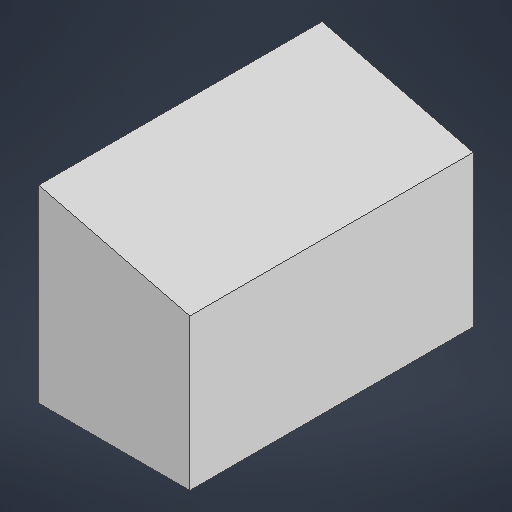
# Autodesk Inventor part: Housing og Buttons & LCD
Saved by Autodesk Inventor 2026.2 (Build 302298010, 298A)
## iProperties
Created: 2026-05-24
Part Number: Housing og Buttons & LCD
Material: Generic
Document SubType Name: Modeling
Designer: lenovo
Density: 1 g/cm^3
Appearance: Default
Author: lenovo
Autodesk Inventor part; units mm, degrees
ref_plane "YZ Plane" through (0, 0, 0) normal (1, 0, 0) x (0, 1, 0)
ref_plane "XZ Plane" through (0, 0, 0) normal (0, 1, 0) x (-1, 0, 0)
ref_plane "XY Plane" through (0, 0, 0) normal (0, 0, 1) x (1, 0, 0)
sketch "Sketch1" plane through (0, 0, 0) normal (0, 0, 1) x (1, 0, 0)
  line L0 (0, 0) -> (80, 0)
  line L1 (0, 0) -> (0, 100)
  line L2 (80, 0) -> (80, 80)
  line L3 (80, 80) -> (0, 100)
  dimension "d0" = 80
  dimension "d1" = 100
  dimension "d2" = 80
  constraints: 8 end point, 1 horizontal, 1 parallel, 1 perpendicular
  measures "d0" distance of L0.start L0.end
  measures "d1" distance of L0.start L1.end
  measures "d2" distance of L0.end L2.end
extrude "Extrusion1" add sketch "Sketch1" along normal blind 150
sketch "Sketch3" plane through (0, 0, 150) normal (0, 0, 1) x (1, 0, 0)
  line L0 (3, 3) -> (3, 96.25)
  line L1 (80, 0) -> (80, 80) projected
  line L2 (77, 3) -> (77, 77.75)
  line L3 (80, 80) -> (0, 100) projected
  line L4 (3, 3) -> (3, 0)
  line L5 (3, 0) -> (77, 0)
  line L6 (77, 0) -> (77, 3)
  line L7 (3, 96.25) -> (77, 77.75)
  point P0 (0, 0)
  dimension "d12" = 93.25
  dimension "d13" = 74
  dimension "d14" = 74.75
  constraints: 12 end point, 2 perpendicular, 2 vertical
  measures "d12" distance of L0.start L0.end
  measures "d13" distance of L0.start L2.start
  measures "d14" distance of L2.start L2.end
extrude "Extrusion3" cut sketch "Sketch3" against normal blind 117
extrude "Extrusion4" add sketch "Sketch3" against normal blind 3
body "Solid1"
